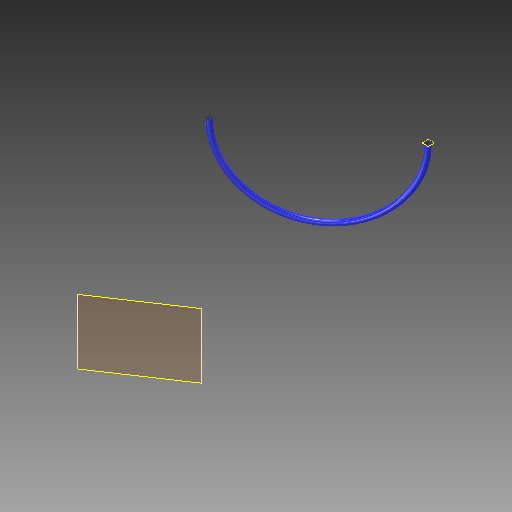
# Autodesk Inventor part: winding_not_formed_3_A
Saved by Autodesk Inventor 2018 (Build 220112000, 112)
## iProperties
Created: 2017-07-07
Part Number: winding_not_formed_3_A
Material: Типовые
Document SubType Name: Modeling
Designer: user
Density: 1 g/cm^3
Appearance: По умолчанию
Author: user
Autodesk Inventor part; units mm, degrees
ref_plane "YZ Plane" through (0, 0, 0) normal (1, 0, 0) x (0, 1, 0)
ref_plane "XZ Plane" through (0, 0, 0) normal (0, 1, 0) x (-1, 0, 0)
ref_plane "XY Plane" through (0, 0, 0) normal (0, 0, 1) x (1, 0, 0)
ref_plane "РабПлоскость1" through (22.2702, 249.9741, -56.4945) normal (0.5555702, 0, 0.8314696) x (0, -1, 0)
sketch "Эскиз2" plane through (22.2702, 249.9741, -56.4945) normal (0.5555702, 0, 0.8314696) x (0, -1, 0)
  arc A0 (0, 0) -> (0, 199.3448) centre (0, 99.6724) ccw
  point P0 (249.9741, -49.9036)
  constraints: 2 point on circle, 1 centre point
ref_plane "РабПлоскость2" through (188.0193, 249.9741, -167.2446) normal (0, -1, 0) x (1, 0, 0)
sketch "Эскиз3" plane through (188.0193, 249.9741, -167.2446) normal (0, -1, 0) x (1, 0, 0)
  circle A0 centre (0, 0) radius 3.5 projected
  circle A1 centre (0, 0) radius 2.5 projected
  point P0 (-188.0193, 167.2446)
sweep "Сдвиг1" add profiles "Эскиз3" path "Эскиз2"
